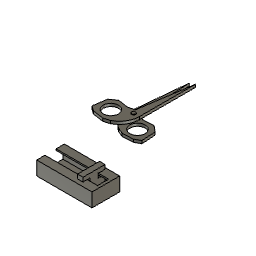
Assembly (Autodesk Fusion 360 design; units mm, degrees)
Autodesk Fusion 360 part; units mm, degrees
note: some values were not read from the file. Set by a fixed rule: which sketch regions a step uses.
sketch "Sketch1" plane through (0, 0, 0) normal (0, 0, 1) x (1, 0, 0)
  line L0 (59.0604, -0.2618) -> (80, -20)
  line L1 (80, -20) -> (80, -70)
  line L2 (80, -70) -> (60, -80)
  line L3 (60, -80) -> (20, -80)
  line L4 (20, -80) -> (0, -70)
  line L5 (-30, 0) -> (0, 200)
  circle A0 centre (38.4073, -40.7325) radius 27.3939
  line L6 (0, 200) -> (0, 10)
  line L7 (0, 10) -> (20, 0)
  line L8 (20, 0) -> (59.0604, -0.2618)
  arc A1 (-30, 0) -> (0, -70) centre (41.6049, -10.7407) ccw
  constraint vertical L1
  constraint horizontal L3
  constraint vertical L6
  constraint tangent L5 A1
extrude "Extrude1" add sketch "Sketch1" along normal blind 10 makes body 1
mirror "Mirror1" about plane through (0, 0, 0) normal (1, 0, 0) of bodies 1 makes body 2
move_body "Move4" bodies 2 to x (0.996195, -0.087156, 0) y (0.087156, 0.996195, 0) z (0, 0, 1) at (-10.1388, -3.5128, 10)
move_body "Move5" bodies 1 to x (0.99863, 0.052336, 0) y (-0.052336, 0.99863, 0) z (0, 0, 1) at (5.4569, -2.5059, 0)
hole "Hole1" at (-0.8281, -8.1517, 20) direction (0, 0, -1) diameter 15 depth 10 tip angle 118 bodies 1 2
sketch "Sketch2" plane through (0, 0, 0) normal (0, 0, -1) x (1, 0, 0)
  circle A0 centre (45.9433, 41.1725) radius 27.3939
  line L0 (-24.502, 4.0759) -> (-5.0103, -197.2201)
  line L1 (-5.0103, -197.2201) -> (4.9335, -7.4804)
  line L2 (4.9335, -7.4804) -> (25.4295, 1.4591)
  line L3 (25.4295, 1.4591) -> (64.45, -0.3237)
  line L4 (64.45, -0.3237) -> (86.394, 18.2916)
  line L5 (86.394, 18.2916) -> (89.0108, 68.223)
  line L6 (89.0108, 68.223) -> (69.5615, 79.2561)
  line L7 (69.5615, 79.2561) -> (29.6164, 81.3495)
  line L8 (29.6164, 81.3495) -> (9.1204, 72.4099)
  arc A1 (9.1204, 72.4099) -> (-24.502, 4.0759) centre (47.5669, 11.0544) ccw
  circle A2 centre (-0.7175, 8.1663) radius 6.6751
extrude "Extrude2" add sketch "Sketch2" against normal blind 22 contours A2 bodies 1
copy_body "Body->Comp1" bodies 1 removing the originals makes body 3 in component "Component"
copy_body "Body->Comp2" bodies 2 removing the originals makes body 4 in component "Component'"
sketch "Sketch3" plane through (0, 0, 0) normal (1, 0, 0) x (0, 1, 0)
  line L0 (-329.8417, 50.1924) -> (-359.8417, 50.1924)
  line L1 (-359.8417, 50.1924) -> (-359.8417, 0.1924)
  line L2 (-359.8417, 0.1924) -> (-259.8417, 0.1924)
  line L3 (-259.8417, 0.1924) -> (-259.8417, 50.1924)
  line L4 (-259.8417, 50.1924) -> (-289.8417, 50.1924)
  line L5 (-289.8417, 50.1924) -> (-289.8417, 45.1924)
  line L6 (-289.8417, 45.1924) -> (-264.8417, 45.1924)
  line L7 (-264.8417, 45.1924) -> (-264.8417, 5.1924)
  line L8 (-264.8417, 5.1924) -> (-354.8417, 5.1924)
  line L9 (-354.8417, 5.1924) -> (-354.8417, 45.1924)
  line L10 (-354.8417, 45.1924) -> (-329.8417, 45.1924)
  line L11 (-329.8417, 45.1924) -> (-329.8417, 50.1924)
  constraint horizontal L0
  constraint perpendicular L0 L1
  constraint perpendicular L1 L2
  constraint perpendicular L2 L3
  constraint perpendicular L3 L4
  constraint perpendicular L4 L5
  constraint perpendicular L5 L6
  constraint perpendicular L6 L7
  constraint perpendicular L7 L8
  constraint perpendicular L8 L9
  constraint perpendicular L9 L10
  constraint perpendicular L10 L11
extrude "Extrude3" add sketch "Sketch3" along normal blind 190 separate body makes body 5
box "BoxPrimitive1" add length 50 width 100 height 10 placed x (0, 0, 1) y (0, -1, 0) z (1, 0, 0) at (190, -259.8417, 0.1924) bodies 5
sketch "Sketch5" plane through (0, 0, 0) normal (-1, 0, 0) x (0, -1, 0)
  line L0 (329.8417, 50.1924) -> (329.8417, 45.1924)
  line L1 (329.8417, 45.1924) -> (354.8417, 45.1924)
  line L2 (354.8417, 45.1924) -> (354.8417, 5.1924)
  line L3 (354.8417, 5.1924) -> (264.8417, 5.1924)
  line L4 (264.8417, 5.1924) -> (264.8417, 45.1924)
  line L5 (264.8417, 45.1924) -> (289.8417, 45.1924)
  line L6 (289.8417, 45.1924) -> (289.8417, 50.1924)
  line L7 (289.8417, 50.1924) -> (259.8417, 50.1924)
  line L8 (259.8417, 50.1924) -> (259.8417, 0.1924)
  line L9 (259.8417, 0.1924) -> (359.8417, 0.1924)
  line L10 (359.8417, 0.1924) -> (359.8417, 50.1924)
  line L11 (359.8417, 50.1924) -> (329.8417, 50.1924)
  line L12 (270, 40) -> (270, 10)
  line L13 (270, 10) -> (350, 10)
  line L14 (350, 10) -> (350, 40)
  line L15 (350, 40) -> (325, 40)
  line L16 (325, 40) -> (325, 55)
  line L17 (325, 55) -> (350, 55)
  line L18 (350, 55) -> (350, 70)
  line L19 (350, 70) -> (270, 70)
  line L20 (270, 70) -> (270, 55)
  line L21 (270, 55) -> (295, 55)
  line L22 (295, 55) -> (295, 40)
  line L23 (295, 40) -> (270, 40)
  constraint parallel L4 L12
  constraint perpendicular L10 L13
  constraint perpendicular L13 L14
  constraint perpendicular L14 L15
  constraint perpendicular L15 L16
  constraint perpendicular L16 L17
  constraint perpendicular L17 L18
  constraint perpendicular L16 L19
  constraint perpendicular L19 L20
  constraint perpendicular L20 L21
  constraint perpendicular L21 L22
  constraint perpendicular L12 L23
extrude "Extrude4" add sketch "Sketch5" against normal blind 20 separate body contours L12 L13 L14 L15 L16 L17 L18 L19 L20 L21 L22 L23 makes body 6
copy_body "Body->Comp3" bodies 6 removing the originals makes body 7 in component "Component''"
copy_body "Body->Comp4" bodies 5 removing the originals makes body 8 in component "Component'''"
component "Component" placed x (1, 0, 0) y (0, 1, 0) z (0, 0, 1) at (0, 0, 0)
component "Component'" placed x (0.998091, -0.061758, 0) y (0.061758, 0.998091, 0) z (0, 0, 1) at (0.2132, -0.0567, 0)
component "Component''" placed x (1, 0, 0) y (0, 1, 0) z (0, 0, 1) at (0, 0, 0)
component "Component'''" placed x (1, 0, 0) y (0, 1, 0) z (0, 0, 1) at (0, 0, 0)
